Autodesk Inventor part; units mm, degrees
(part 2 of 3)
  point P0 (100, -8.64)
  point P1 (128.2327, 105.01)
  point P2 (153.2327, 105.01)
  point P3 (180, 101.1463)
  point P4 (178.2327, 105.01)
  point P5 (103.2327, 105.01)
  point P6 (8.5673, 105.01)
  point P7 (78.2327, 105.01)
  point P8 (53.2327, 105.01)
  point P9 (28.2327, 105.01)
  point P10 (128.2327, 105.01)
  point P11 (153.2327, 105.01)
  point P12 (178.2327, 105.01)
  point P13 (103.2327, 105.01)
  point P14 (78.2327, 105.01)
  point P15 (53.2327, 105.01)
  point P16 (28.2327, 105.01)
  point P17 (3.2779, 105.049)
  point P18 (3.2327, 105.01)
  point P19 (8.5221, 105.049)
  dimension "d96" = 1.8
  dimension "d97" = 0.9
  dimension "d100" = 25
  constraints: 98 end point, 82 point on circle, 32 centre point, 8 symmetric about line, 2 coincident, 1 horizontal, 1 vertical, 220 other
  measures "d96" distance between parallel lines of L3 L1
  measures "d97" distance between parallel lines of L115 L111
  measures "d100" distance of L0.end L120.start
extrude "Wyciągnięcie proste7" cut sketch "Szkic8" against normal up to surface (1.2 mm away) contours L0 L1 A0 L110 A1 | A3 L116 A2 L3 L4 | L12 L11 A6 L122 A7 | A8 L123 A9 L9 L8 | L33 L32 A10 L128 A11 | A32 L159 A33 L57 L56 | A12 L129 A13 L30 L29 | L55 L54 A14 L134 A15 | L60 L59 A30 L158 A31 | A28 L153 A29 L62 L61 | A16 L135 A17 L52 L51 | L69 L70 A18 L140 A19 | L65 L64 A26 L152 A27 | A24 L147 A25 L46 L47 | A20 L141 A21 L72 L73 | L43 L44 A22 L146 A23
sketch "Szkic9" plane through (-110, 55, 0) normal (0, 1, 0) x (1, 0, 0)
  line L0 (66.3974, -14.0224) -> (153.6026, -14.0224) construction
  line L1 (153.6026, -14.0224) -> (153.6026, -101.2276) construction
  line L2 (153.6026, -101.2276) -> (66.3974, -101.2276) construction
  line L3 (66.3974, -101.2276) -> (66.3974, -14.0224) construction
  line L4 (0, 0) -> (0, -115.25) projected
  line L5 (220, 0) -> (220, -115.25) projected
  line L6 (220, 0) -> (0, 0) projected
  line L7 (220, -115.25) -> (0, -115.25) projected
  point P0 (110, 0)
  dimension "d115" = 66.3975
  dimension "d117" = 87.2051
  dimension "d118" = 220
  dimension "d121" = 115.25
  dimension "d122" = 87.2051
  dimension "d123" = 14.0224
  constraints: 2 other
  measures "d115" distance between parallel lines of L4 L3
  measures "d117" distance between parallel lines of L1 L3
  measures "d118" distance between parallel lines of L5 L4
  measures "d121" distance between parallel lines of L6 L7
  measures "d122" distance between parallel lines of L0 L2
  measures "d123" distance between parallel lines of L6 L0
decal "Pokrycie bitmapą1"
ref_plane "Płaszczyzna konstrukcyjna8" through (-110, 55, 0) normal (0, 1, 0) x (1, 0, 0)
sketch "Szkic13" plane through (-110, 55, 0) normal (0, 1, 0) x (1, 0, 0)
  spline S0 degree 3 poles (103.4764, -89.9857) (102.0188, -89.9857) (101.1686, -88.8719) (101.1686, -87.4139) (101.1686, -85.9559) (102.0188, -84.8422) (103.4764, -84.8422) (104.9341, -84.8422) (105.7843, -85.9559) (105.7843, -87.4139) (105.7843, -88.8719) (104.9341, -89.9857) (103.4764, -89.9857) knots 0 0 0 0 0.25 0.25 0.25 0.5 0.5 0.5 0.75 0.75 0.75 1 1 1 1
  line L0 (103.4764, -89.9857) -> (102.0188, -89.9857) construction
  line L1 (102.0188, -89.9857) -> (101.1686, -88.8719) construction
  line L2 (101.1686, -88.8719) -> (101.1686, -87.4139) construction
  line L3 (101.1686, -87.4139) -> (101.1686, -85.9559) construction
  line L4 (101.1686, -85.9559) -> (102.0188, -84.8422) construction
  line L5 (102.0188, -84.8422) -> (103.4764, -84.8422) construction
  line L6 (103.4764, -84.8422) -> (104.9341, -84.8422) construction
  line L7 (104.9341, -84.8422) -> (105.7843, -85.9559) construction
  line L8 (105.7843, -85.9559) -> (105.7843, -87.4139) construction
  line L9 (105.7843, -87.4139) -> (105.7843, -88.8719) construction
  line L10 (105.7843, -88.8719) -> (104.9341, -89.9857) construction
  line L11 (104.9341, -89.9857) -> (103.4764, -89.9857) construction
  spline S1 degree 3 poles (105.7843, -83.3845) (105.096, -82.7766) (104.2254, -82.3921) (103.1727, -82.3921) (100.3586, -82.3921) (98.5368, -84.5991) (98.5368, -87.4139) (98.5368, -90.2284) (100.3586, -92.4562) (103.1727, -92.4562) (104.2254, -92.4562) (105.096, -92.0713) (105.7843, -91.4638) knots 0 0 0 0 0.111111 0.111111 0.111111 0.222222 0.222222 0.222222 0.333333 0.333333 0.333333 0.444444 0.444444 0.444444 0.444444
  line L12 (105.7843, -83.3845) -> (105.096, -82.7766) construction
  line L13 (105.096, -82.7766) -> (104.2254, -82.3921) construction
  line L14 (104.2254, -82.3921) -> (103.1727, -82.3921) construction
  line L15 (103.1727, -82.3921) -> (100.3586, -82.3921) construction
  line L16 (100.3586, -82.3921) -> (98.5368, -84.5991) construction
  line L17 (98.5368, -84.5991) -> (98.5368, -87.4139) construction
  line L18 (98.5368, -87.4139) -> (98.5368, -90.2284) construction
  line L19 (98.5368, -90.2284) -> (100.3586, -92.4562) construction
  line L20 (100.3586, -92.4562) -> (103.1727, -92.4562) construction
  line L21 (103.1727, -92.4562) -> (104.2254, -92.4562) construction
  line L22 (104.2254, -92.4562) -> (105.096, -92.0713) construction
  line L23 (105.096, -92.0713) -> (105.7843, -91.4638) construction
  line L24 (105.7843, -91.4638) -> (105.7843, -92.2939)
  line L25 (105.7843, -92.2939) -> (108.4767, -92.2939)
  line L26 (108.4767, -92.2939) -> (108.4767, -78.1196)
  line L27 (108.4767, -78.1196) -> (105.7843, -78.1196)
  line L28 (105.7843, -78.1196) -> (105.7843, -83.3845)
  spline S2 degree 3 poles (152.4794, -86.3203) (150.9406, -85.8546) (150.6576, -85.6119) (150.6372, -85.2471) knots 0 0 0 0 0.071429 0.071429 0.071429 0.071429
  line L29 (152.4794, -86.3203) -> (150.9406, -85.8546) construction
  line L30 (150.9406, -85.8546) -> (150.6576, -85.6119) construction
  line L31 (150.6576, -85.6119) -> (150.6372, -85.2471) construction
  spline S3 degree 3 poles (150.6372, -85.2471) (150.6167, -84.984) (150.8802, -84.4781) (151.9125, -84.5589) knots 0.071429 0.071429 0.071429 0.071429 0.142857 0.142857 0.142857 0.142857
  line L32 (150.6372, -85.2471) -> (150.6167, -84.984) construction
  line L33 (150.6167, -84.984) -> (150.8802, -84.4781) construction
  line L34 (150.8802, -84.4781) -> (151.9125, -84.5589) construction
  spline S4 degree 3 poles (151.9125, -84.5589) (152.6614, -84.6195) (152.9853, -85.0852) (153.0865, -85.4091) knots 0.142857 0.142857 0.142857 0.142857 0.214286 0.214286 0.214286 0.214286
  line L35 (151.9125, -84.5589) -> (152.6614, -84.6195) construction
  line L36 (152.6614, -84.6195) -> (152.9853, -85.0852) construction
  line L37 (152.9853, -85.0852) -> (153.0865, -85.4091) construction
  line L38 (153.0865, -85.4091) -> (155.1517, -84.822)
  spline S5 degree 3 poles (155.1517, -84.822) (155.0102, -83.9313) (153.8965, -82.4122) (151.5481, -82.4122) (149.0176, -82.4122) (147.9243, -83.83) (147.8636, -85.1865) knots 0.285714 0.285714 0.285714 0.285714 0.357143 0.357143 0.357143 0.428571 0.428571 0.428571 0.428571
  line L39 (155.1517, -84.822) -> (155.0102, -83.9313) construction
  line L40 (155.0102, -83.9313) -> (153.8965, -82.4122) construction
  line L41 (153.8965, -82.4122) -> (151.5481, -82.4122) construction
  line L42 (151.5481, -82.4122) -> (149.0176, -82.4122) construction
  line L43 (149.0176, -82.4122) -> (147.9243, -83.83) construction
  line L44 (147.9243, -83.83) -> (147.8636, -85.1865) construction
  spline S6 degree 3 poles (147.8636, -85.1865) (147.803, -86.7863) (148.7343, -87.5151) (150.8598, -88.2644) knots 0.428571 0.428571 0.428571 0.428571 0.5 0.5 0.5 0.5
  line L45 (147.8636, -85.1865) -> (147.803, -86.7863) construction
  line L46 (147.803, -86.7863) -> (148.7343, -87.5151) construction
  line L47 (148.7343, -87.5151) -> (150.8598, -88.2644) construction
  spline S7 degree 3 poles (150.8598, -88.2644) (152.2162, -88.7301) (152.6819, -88.7908) (152.7023, -89.3376) knots 0.5 0.5 0.5 0.5 0.571429 0.571429 0.571429 0.571429
  line L48 (150.8598, -88.2644) -> (152.2162, -88.7301) construction
  line L49 (152.2162, -88.7301) -> (152.6819, -88.7908) construction
  line L50 (152.6819, -88.7908) -> (152.7023, -89.3376) construction
  spline S8 degree 3 poles (152.7023, -89.3376) (152.7221, -89.8639) (151.9125, -90.0463) (151.1836, -90.0061) knots 0.571429 0.571429 0.571429 0.571429 0.642857 0.642857 0.642857 0.642857
  line L51 (152.7023, -89.3376) -> (152.7221, -89.8639) construction
  line L52 (152.7221, -89.8639) -> (151.9125, -90.0463) construction
  line L53 (151.9125, -90.0463) -> (151.1836, -90.0061) construction
  spline S9 degree 3 poles (151.1836, -90.0061) (150.4954, -89.9652) (149.6452, -89.5606) (149.4427, -89.054) knots 0.642857 0.642857 0.642857 0.642857 0.714286 0.714286 0.714286 0.714286
  line L54 (151.1836, -90.0061) -> (150.4954, -89.9652) construction
  line L55 (150.4954, -89.9652) -> (149.6452, -89.5606) construction
  line L56 (149.6452, -89.5606) -> (149.4427, -89.054) construction
  line L57 (149.4427, -89.054) -> (147.4788, -90.1074)
  spline S10 degree 3 poles (147.4788, -90.1074) (147.803, -91.3015) (149.6046, -92.4357) (151.6493, -92.4357) (153.8965, -92.4357) (155.4755, -91.2412) (155.5366, -89.4791) knots 0.785714 0.785714 0.785714 0.785714 0.857143 0.857143 0.857143 0.928571 0.928571 0.928571 0.928571
  line L58 (147.4788, -90.1074) -> (147.803, -91.3015) construction
  line L59 (147.803, -91.3015) -> (149.6046, -92.4357) construction
  line L60 (149.6046, -92.4357) -> (151.6493, -92.4357) construction
  line L61 (151.6493, -92.4357) -> (153.8965, -92.4357) construction
  line L62 (153.8965, -92.4357) -> (155.4755, -91.2412) construction
  line L63 (155.4755, -91.2412) -> (155.5366, -89.4791) construction
  spline S11 degree 3 poles (155.5366, -89.4791) (155.5972, -88.0013) (154.7672, -87.029) (152.4794, -86.3203) knots 0.928571 0.928571 0.928571 0.928571 1 1 1 1
  line L64 (155.5366, -89.4791) -> (155.5972, -88.0013) construction
  line L65 (155.5972, -88.0013) -> (154.7672, -87.029) construction
  line L66 (154.7672, -87.029) -> (152.4794, -86.3203) construction
  spline S12 degree 3 poles (141.9948, -89.9857) (140.5372, -89.9857) (139.6866, -88.8719) (139.6866, -87.4139) (139.6866, -85.9559) (140.5372, -84.8422) (141.9948, -84.8422) (143.4321, -84.8422) (144.2822, -85.9559) (144.2822, -87.4139) (144.2822, -88.8719) (143.4321, -89.9857) (141.9948, -89.9857) knots 0 0 0 0 0.25 0.25 0.25 0.5 0.5 0.5 0.75 0.75 0.75 1 1 1 1
  line L67 (141.9948, -89.9857) -> (140.5372, -89.9857) construction
  line L68 (140.5372, -89.9857) -> (139.6866, -88.8719) construction
  line L69 (139.6866, -88.8719) -> (139.6866, -87.4139) construction
  line L70 (139.6866, -87.4139) -> (139.6866, -85.9559) construction
  line L71 (139.6866, -85.9559) -> (140.5372, -84.8422) construction
  line L72 (140.5372, -84.8422) -> (141.9948, -84.8422) construction
  line L73 (141.9948, -84.8422) -> (143.4321, -84.8422) construction
  line L74 (143.4321, -84.8422) -> (144.2822, -85.9559) construction
  line L75 (144.2822, -85.9559) -> (144.2822, -87.4139) construction
  line L76 (144.2822, -87.4139) -> (144.2822, -88.8719) construction
  line L77 (144.2822, -88.8719) -> (143.4321, -89.9857) construction
  line L78 (143.4321, -89.9857) -> (141.9948, -89.9857) construction
  spline S13 degree 3 poles (142.2781, -82.3921) (141.2455, -82.3921) (140.3551, -82.7766) (139.6866, -83.3845) knots 0 0 0 0 0.111111 0.111111 0.111111 0.111111
  line L79 (142.2781, -82.3921) -> (141.2455, -82.3921) construction
  line L80 (141.2455, -82.3921) -> (140.3551, -82.7766) construction
  line L81 (140.3551, -82.7766) -> (139.6866, -83.3845) construction
  line L82 (139.6866, -83.3845) -> (139.6866, -78.1196)
  line L83 (139.6866, -78.1196) -> (136.9942, -78.1196)
  line L84 (136.9942, -78.1196) -> (136.9942, -92.2939)
  line L85 (136.9942, -92.2939) -> (139.6866, -92.2939)
  line L86 (139.6866, -92.2939) -> (139.6866, -91.4638)
  spline S14 degree 3 poles (139.6866, -91.4638) (140.3551, -92.0713) (141.2455, -92.4562) (142.2781, -92.4562) (145.0922, -92.4562) (146.9746, -90.2284) (146.9746, -87.4139) (146.9746, -84.5991) (145.0922, -82.3921) (142.2781, -82.3921) knots 0.666667 0.666667 0.666667 0.666667 0.777778 0.777778 0.777778 0.888889 0.888889 0.888889 1 1 1 1
  line L87 (139.6866, -91.4638) -> (140.3551, -92.0713) construction
  line L88 (140.3551, -92.0713) -> (141.2455, -92.4562) construction
  line L89 (141.2455, -92.4562) -> (142.2781, -92.4562) construction
  line L90 (142.2781, -92.4562) -> (145.0922, -92.4562) construction
  line L91 (145.0922, -92.4562) -> (146.9746, -90.2284) construction
  line L92 (146.9746, -90.2284) -> (146.9746, -87.4139) construction
  line L93 (146.9746, -87.4139) -> (146.9746, -84.5991) construction
  line L94 (146.9746, -84.5991) -> (145.0922, -82.3921) construction
  line L95 (145.0922, -82.3921) -> (142.2781, -82.3921) construction
  spline S15 degree 3 poles (123.5872, -89.9652) (122.8584, -89.9049) (122.6965, -89.1757) (122.6965, -88.5075) knots 0 0 0 0 0.125 0.125 0.125 0.125
  line L96 (123.5872, -89.9652) -> (122.8584, -89.9049) construction
  line L97 (122.8584, -89.9049) -> (122.6965, -89.1757) construction
  line L98 (122.6965, -89.1757) -> (122.6965, -88.5075) construction
  line L99 (122.6965, -88.5075) -> (122.6965, -77.1071)
  line L100 (122.6965, -77.1071) -> (120.0037, -77.1071)
  line L101 (120.0037, -77.1071) -> (120.0037, -88.3657)
  spline S16 degree 3 poles (120.0037, -88.3657) (120.0037, -91.6056) (121.2593, -92.375) (122.9191, -92.4562) knots 0.5 0.5 0.5 0.5 0.625 0.625 0.625 0.625
  line L102 (120.0037, -88.3657) -> (120.0037, -91.6056) construction
  line L103 (120.0037, -91.6056) -> (121.2593, -92.375) construction
  line L104 (121.2593, -92.375) -> (122.9191, -92.4562) construction
  spline S17 degree 3 poles (122.9191, -92.4562) (124.0935, -92.5168) (125.8125, -92.36) (125.8143, -92.3598) knots 0.625 0.625 0.625 0.625 0.75 0.75 0.75 0.75
  line L105 (122.9191, -92.4562) -> (124.0935, -92.5168) construction
  line L106 (124.0935, -92.5168) -> (125.8143, -92.3598) construction
  line L107 (125.8143, -92.3598) -> (125.8143, -92.3598) construction
  line L108 (125.8143, -92.3598) -> (125.6171, -89.9941)
  spline S18 degree 3 poles (125.6171, -89.9941) (125.6155, -89.9942) (124.0123, -90.0061) (123.5872, -89.9652) knots 0.875 0.875 0.875 0.875 1 1 1 1
  line L109 (125.6171, -89.9941) -> (125.6171, -89.9941) construction
  line L110 (125.6171, -89.9941) -> (124.0123, -90.0061) construction
  line L111 (124.0123, -90.0061) -> (123.5872, -89.9652) construction
  spline S19 degree 3 poles (112.443, -86.5027) (112.6857, -85.5308) (113.3944, -84.8422) (114.5283, -84.8422) (115.6617, -84.8422) (116.2689, -85.5308) (116.4918, -86.5027) knots 0 0 0 0 0.333333 0.333333 0.333333 0.666667 0.666667 0.666667 0.666667
  line L112 (112.443, -86.5027) -> (112.6857, -85.5308) construction
  line L113 (112.6857, -85.5308) -> (113.3944, -84.8422) construction
  line L114 (113.3944, -84.8422) -> (114.5283, -84.8422) construction
  line L115 (114.5283, -84.8422) -> (115.6617, -84.8422) construction
  line L116 (115.6617, -84.8422) -> (116.2689, -85.5308) construction
  line L117 (116.2689, -85.5308) -> (116.4918, -86.5027) construction
  line L118 (116.4918, -86.5027) -> (112.443, -86.5027)
  spline S20 degree 3 poles (114.5283, -82.3921) (111.7138, -82.3921) (109.6896, -84.5991) (109.6896, -87.4139) (109.6896, -90.2284) (111.815, -92.4562) (114.6292, -92.4562) (116.411, -92.4562) (117.8483, -91.565) (118.6579, -90.2083) knots 0 0 0 0 0.111111 0.111111 0.111111 0.222222 0.222222 0.222222 0.333333 0.333333 0.333333 0.333333
  line L119 (114.5283, -82.3921) -> (111.7138, -82.3921) construction
  line L120 (111.7138, -82.3921) -> (109.6896, -84.5991) construction
  line L121 (109.6896, -84.5991) -> (109.6896, -87.4139) construction
  line L122 (109.6896, -87.4139) -> (109.6896, -90.2284) construction
  line L123 (109.6896, -90.2284) -> (111.815, -92.4562) construction
  line L124 (111.815, -92.4562) -> (114.6292, -92.4562) construction
  line L125 (114.6292, -92.4562) -> (116.411, -92.4562) construction
  line L126 (116.411, -92.4562) -> (117.8483, -91.565) construction
  line L127 (117.8483, -91.565) -> (118.6579, -90.2083) construction
  line L128 (118.6579, -90.2083) -> (116.4308, -89.1146)
  spline S21 degree 3 poles (116.4308, -89.1146) (116.0463, -89.6614) (115.4187, -89.9857) (114.6292, -89.9857) (113.5158, -89.9857) (112.7665, -89.3376) (112.4631, -88.3858) knots 0.444444 0.444444 0.444444 0.444444 0.555556 0.555556 0.555556 0.666667 0.666667 0.666667 0.666667
  line L129 (116.4308, -89.1146) -> (116.0463, -89.6614) construction
  line L130 (116.0463, -89.6614) -> (115.4187, -89.9857) construction
  line L131 (115.4187, -89.9857) -> (114.6292, -89.9857) construction
  line L132 (114.6292, -89.9857) -> (113.5158, -89.9857) construction
  line L133 (113.5158, -89.9857) -> (112.7665, -89.3376) construction
  line L134 (112.7665, -89.3376) -> (112.4631, -88.3858) construction
  line L135 (112.4631, -88.3858) -> (118.9616, -88.3858)
  spline S22 degree 3 poles (118.9616, -88.3858) (119.0223, -88.0821) (119.0428, -87.7582) (119.0428, -87.4139) (119.0428, -84.5991) (117.3219, -82.3921) (114.5283, -82.3921) knots 0.777778 0.777778 0.777778 0.777778 0.888889 0.888889 0.888889 1 1 1 1
  line L136 (118.9616, -88.3858) -> (119.0223, -88.0821) construction
  line L137 (119.0223, -88.0821) -> (119.0428, -87.7582) construction
  line L138 (119.0428, -87.7582) -> (119.0428, -87.4139) construction
  line L139 (119.0428, -87.4139) -> (119.0428, -84.5991) construction
  line L140 (119.0428, -84.5991) -> (117.3219, -82.3921) construction
  line L141 (117.3219, -82.3921) -> (114.5283, -82.3921) construction
  spline S23 degree 3 poles (83.196, -88.3047) (83.1148, -89.3782) (82.3659, -90.2083) (81.3132, -90.3705) knots 0 0 0 0 0.2 0.2 0.2 0.2
  line L142 (83.196, -88.3047) -> (83.1148, -89.3782) construction
  line L143 (83.1148, -89.3782) -> (82.3659, -90.2083) construction
  line L144 (82.3659, -90.2083) -> (81.3132, -90.3705) construction
  spline S24 degree 3 poles (81.3132, -90.3705) (80.7057, -90.4718) (80.0982, -90.3501) (79.9363, -89.9049) knots 0.2 0.2 0.2 0.2 0.4 0.4 0.4 0.4
  line L145 (81.3132, -90.3705) -> (80.7057, -90.4718) construction
  line L146 (80.7057, -90.4718) -> (80.0982, -90.3501) construction
  line L147 (80.0982, -90.3501) -> (79.9363, -89.9049) construction
  spline S25 degree 3 poles (79.9363, -89.9049) (79.7543, -89.4187) (80.0375, -88.7707) (81.0295, -88.5075) knots 0.4 0.4 0.4 0.4 0.6 0.6 0.6 0.6
  line L148 (79.9363, -89.9049) -> (79.7543, -89.4187) construction
  line L149 (79.7543, -89.4187) -> (80.0375, -88.7707) construction
  line L150 (80.0375, -88.7707) -> (81.0295, -88.5075) construction
  spline S26 degree 3 poles (81.0295, -88.5075) (82.3048, -88.1837) (83.1951, -88.0015) (83.196, -88.0013) knots 0.6 0.6 0.6 0.6 0.8 0.8 0.8 0.8
  line L151 (81.0295, -88.5075) -> (82.3048, -88.1837) construction
  line L152 (82.3048, -88.1837) -> (83.196, -88.0013) construction
  line L153 (83.196, -88.0013) -> (83.196, -88.0013) construction
  line L154 (83.196, -88.0013) -> (83.196, -88.3047)
  spline S27 degree 3 poles (81.8797, -82.3921) (79.4505, -82.3921) (78.0129, -83.992) (77.8309, -85.2676) knots 0 0 0 0 0.083333 0.083333 0.083333 0.083333
  line L155 (81.8797, -82.3921) -> (79.4505, -82.3921) construction
  line L156 (79.4505, -82.3921) -> (78.0129, -83.992) construction
  line L157 (78.0129, -83.992) -> (77.8309, -85.2676) construction
  line L158 (77.8309, -85.2676) -> (80.0781, -85.7537)
  spline S28 degree 3 poles (80.0781, -85.7537) (80.24, -85.0044) (80.8676, -84.6195) (81.6977, -84.5991) knots 0.166667 0.166667 0.166667 0.166667 0.25 0.25 0.25 0.25
  line L159 (80.0781, -85.7537) -> (80.24, -85.0044) construction
  line L160 (80.24, -85.0044) -> (80.8676, -84.6195) construction
  line L161 (80.8676, -84.6195) -> (81.6977, -84.5991) construction
  spline S29 degree 3 poles (81.6977, -84.5991) (82.6491, -84.5589) (83.2767, -85.1664) (83.1349, -85.7537) knots 0.25 0.25 0.25 0.25 0.333333 0.333333 0.333333 0.333333
  line L162 (81.6977, -84.5991) -> (82.6491, -84.5589) construction
  line L163 (82.6491, -84.5589) -> (83.2767, -85.1664) construction
  line L164 (83.2767, -85.1664) -> (83.1349, -85.7537) construction
  spline S30 degree 3 poles (83.1349, -85.7537) (83.0136, -86.3002) (82.3253, -86.3002) (80.6856, -86.6646) knots 0.333333 0.333333 0.333333 0.333333 0.416667 0.416667 0.416667 0.416667
  line L165 (83.1349, -85.7537) -> (83.0136, -86.3002) construction
  line L166 (83.0136, -86.3002) -> (82.3253, -86.3002) construction
  line L167 (82.3253, -86.3002) -> (80.6856, -86.6646) construction
  spline S31 degree 3 poles (80.6856, -86.6646) (78.6204, -87.1105) (77.1627, -87.8595) (77.1627, -89.9857) knots 0.416667 0.416667 0.416667 0.416667 0.5 0.5 0.5 0.5
  line L168 (80.6856, -86.6646) -> (78.6204, -87.1105) construction
  line L169 (78.6204, -87.1105) -> (77.1627, -87.8595) construction
  line L170 (77.1627, -87.8595) -> (77.1627, -89.9857) construction
  spline S32 degree 3 poles (77.1627, -89.9857) (77.2439, -91.4638) (78.2966, -92.4562) (80.1995, -92.4562) (81.8596, -92.4562) (82.8315, -91.7471) (83.196, -91.3827) knots 0.5 0.5 0.5 0.5 0.583333 0.583333 0.583333 0.666667 0.666667 0.666667 0.666667
  line L171 (77.1627, -89.9857) -> (77.2439, -91.4638) construction
  line L172 (77.2439, -91.4638) -> (78.2966, -92.4562) construction
  line L173 (78.2966, -92.4562) -> (80.1995, -92.4562) construction
  line L174 (80.1995, -92.4562) -> (81.8596, -92.4562) construction
  line L175 (81.8596, -92.4562) -> (82.8315, -91.7471) construction
  line L176 (82.8315, -91.7471) -> (83.196, -91.3827) construction
  line L177 (83.196, -91.3827) -> (83.196, -92.2939)
  line L178 (83.196, -92.2939) -> (85.8679, -92.2939)
  line L179 (85.8679, -92.2939) -> (85.8679, -86.1993)
  spline S33 degree 3 poles (85.8679, -86.1993) (85.8679, -83.364) (84.0056, -82.3921) (81.8797, -82.3921) knots 0.916667 0.916667 0.916667 0.916667 1 1 1 1
  line L180 (85.8679, -86.1993) -> (85.8679, -83.364) construction
  line L181 (85.8679, -83.364) -> (84.0056, -82.3921) construction
  line L182 (84.0056, -82.3921) -> (81.8797, -82.3921) construction
  line L183 (73.1478, -83.8678) -> (67.5033, -83.8678)
  line L184 (67.5033, -83.8678) -> (67.5033, -78.2233)
  line L185 (67.5033, -78.2233) -> (64.6811, -78.2233)
  line L186 (64.6811, -78.2233) -> (64.6811, -83.8678)
  line L187 (64.6811, -83.8678) -> (64.6811, -86.69)
  line L188 (64.6811, -86.69) -> (64.6811, -92.3344)
  line L189 (64.6811, -92.3344) -> (67.5033, -92.3344)
  line L190 (67.5033, -92.3344) -> (67.5033, -86.69)
  line L191 (67.5033, -86.69) -> (73.1478, -86.69)
  line L192 (73.1478, -86.69) -> (73.1478, -92.3344)
  line L193 (73.1478, -92.3344) -> (75.97, -92.3344)
  line L194 (75.97, -92.3344) -> (75.97, -86.69)
  line L195 (75.97, -86.69) -> (75.97, -83.8678)
  line L196 (75.97, -83.8678) -> (75.97, -78.2233)
  line L197 (75.97, -78.2233) -> (73.1478, -78.2233)
  line L198 (73.1478, -78.2233) -> (73.1478, -83.8678)
  spline S34 degree 3 poles (132.7041, -88.3047) (132.6233, -89.3782) (131.8743, -90.2083) (130.8213, -90.3705) knots 0 0 0 0 0.2 0.2 0.2 0.2
  line L199 (132.7041, -88.3047) -> (132.6233, -89.3782) construction
  line L200 (132.6233, -89.3782) -> (131.8743, -90.2083) construction
  line L201 (131.8743, -90.2083) -> (130.8213, -90.3705) construction
  spline S35 degree 3 poles (130.8213, -90.3705) (130.2142, -90.4718) (129.6067, -90.3501) (129.4448, -89.9049) knots 0.2 0.2 0.2 0.2 0.4 0.4 0.4 0.4
  line L202 (130.8213, -90.3705) -> (130.2142, -90.4718) construction
  line L203 (130.2142, -90.4718) -> (129.6067, -90.3501) construction
  line L204 (129.6067, -90.3501) -> (129.4448, -89.9049) construction
  spline S36 degree 3 poles (129.4448, -89.9049) (129.2627, -89.4187) (129.546, -88.7707) (130.538, -88.5075) knots 0.4 0.4 0.4 0.4 0.6 0.6 0.6 0.6
  line L205 (129.4448, -89.9049) -> (129.2627, -89.4187) construction
  line L206 (129.2627, -89.4187) -> (129.546, -88.7707) construction
  line L207 (129.546, -88.7707) -> (130.538, -88.5075) construction
  spline S37 degree 3 poles (130.538, -88.5075) (131.8137, -88.1837) (132.7032, -88.0015) (132.7041, -88.0013) knots 0.6 0.6 0.6 0.6 0.8 0.8 0.8 0.8
  line L208 (130.538, -88.5075) -> (131.8137, -88.1837) construction
  line L209 (131.8137, -88.1837) -> (132.7041, -88.0013) construction
  line L210 (132.7041, -88.0013) -> (132.7041, -88.0013) construction
  line L211 (132.7041, -88.0013) -> (132.7041, -88.3047)
  spline S38 degree 3 poles (131.3886, -82.3921) (128.959, -82.3921) (127.5218, -83.992) (127.3394, -85.2676) knots 0 0 0 0 0.083333 0.083333 0.083333 0.083333
  line L212 (131.3886, -82.3921) -> (128.959, -82.3921) construction
  line L213 (128.959, -82.3921) -> (127.5218, -83.992) construction
  line L214 (127.5218, -83.992) -> (127.3394, -85.2676) construction
  line L215 (127.3394, -85.2676) -> (129.5866, -85.7537)
  spline S39 degree 3 poles (129.5866, -85.7537) (129.7485, -85.0044) (130.3761, -84.6195) (131.2062, -84.5991) knots 0.166667 0.166667 0.166667 0.166667 0.25 0.25 0.25 0.25
  line L216 (129.5866, -85.7537) -> (129.7485, -85.0044) construction
  line L217 (129.7485, -85.0044) -> (130.3761, -84.6195) construction
  line L218 (130.3761, -84.6195) -> (131.2062, -84.5991) construction
  spline S40 degree 3 poles (131.2062, -84.5991) (132.1576, -84.5589) (132.7852, -85.1664) (132.6434, -85.7537) knots 0.25 0.25 0.25 0.25 0.333333 0.333333 0.333333 0.333333
  line L219 (131.2062, -84.5991) -> (132.1576, -84.5589) construction
  line L220 (132.1576, -84.5589) -> (132.7852, -85.1664) construction
  line L221 (132.7852, -85.1664) -> (132.6434, -85.7537) construction
  spline S41 degree 3 poles (132.6434, -85.7537) (132.522, -86.3002) (131.8338, -86.3002) (130.1941, -86.6646) knots 0.333333 0.333333 0.333333 0.333333 0.416667 0.416667 0.416667 0.416667
  line L222 (132.6434, -85.7537) -> (132.522, -86.3002) construction
  line L223 (132.522, -86.3002) -> (131.8338, -86.3002) construction
  line L224 (131.8338, -86.3002) -> (130.1941, -86.6646) construction
  spline S42 degree 3 poles (130.1941, -86.6646) (128.1289, -87.1105) (126.6716, -87.8595) (126.6716, -89.9857) knots 0.416667 0.416667 0.416667 0.416667 0.5 0.5 0.5 0.5
  line L225 (130.1941, -86.6646) -> (128.1289, -87.1105) construction
  line L226 (128.1289, -87.1105) -> (126.6716, -87.8595) construction
  line L227 (126.6716, -87.8595) -> (126.6716, -89.9857) construction
  spline S43 degree 3 poles (126.6716, -89.9857) (126.7524, -91.4638) (127.8047, -92.4562) (129.7079, -92.4562) (131.3681, -92.4562) (132.34, -91.7471) (132.7041, -91.3827) knots 0.5 0.5 0.5 0.5 0.583333 0.583333 0.583333 0.666667 0.666667 0.666667 0.666667
  line L228 (126.6716, -89.9857) -> (126.7524, -91.4638) construction
  line L229 (126.7524, -91.4638) -> (127.8047, -92.4562) construction
  line L230 (127.8047, -92.4562) -> (129.7079, -92.4562) construction
  line L231 (129.7079, -92.4562) -> (131.3681, -92.4562) construction
  line L232 (131.3681, -92.4562) -> (132.34, -91.7471) construction
  line L233 (132.34, -91.7471) -> (132.7041, -91.3827) construction
  line L234 (132.7041, -91.3827) -> (132.7041, -92.2939)
  line L235 (132.7041, -92.2939) -> (135.3764, -92.2939)
  line L236 (135.3764, -92.2939) -> (135.3764, -86.1993)
  spline S44 degree 3 poles (135.3764, -86.1993) (135.3764, -83.364) (133.5141, -82.3921) (131.3886, -82.3921) knots 0.916667 0.916667 0.916667 0.916667 1 1 1 1
  line L237 (135.3764, -86.1993) -> (135.3764, -83.364) construction
  line L238 (135.3764, -83.364) -> (133.5141, -82.3921) construction
  line L239 (133.5141, -82.3921) -> (131.3886, -82.3921) construction
  line L240 (94.4683, -92.2939) -> (97.161, -92.2939)
  line L241 (97.161, -92.2939) -> (97.161, -82.5339)
  line L242 (97.161, -82.5339) -> (94.4683, -82.5339)
  line L243 (94.4683, -82.5339) -> (94.4683, -92.2939)
  spline S45 degree 3 poles (95.825, -78.1602) (94.9745, -78.1602) (94.3063, -78.8283) (94.3063, -79.6785) (94.3063, -80.509) (94.9745, -81.1771) (95.825, -81.1771) (96.6551, -81.1771) (97.3229, -80.509) (97.3229, -79.6785) (97.3229, -78.8283) (96.6551, -78.1602) (95.825, -78.1602) knots 0 0 0 0 0.25 0.25 0.25 0.5 0.5 0.5 0.75 0.75 0.75 1 1 1 1
  line L244 (95.825, -78.1602) -> (94.9745, -78.1602) construction
  line L245 (94.9745, -78.1602) -> (94.3063, -78.8283) construction
  line L246 (94.3063, -78.8283) -> (94.3063, -79.6785) construction
  line L247 (94.3063, -79.6785) -> (94.3063, -80.509) construction
  line L248 (94.3063, -80.509) -> (94.9745, -81.1771) construction
  line L249 (94.9745, -81.1771) -> (95.825, -81.1771) construction
  line L250 (95.825, -81.1771) -> (96.6551, -81.1771) construction
  line L251 (96.6551, -81.1771) -> (97.3229, -80.509) construction
  line L252 (97.3229, -80.509) -> (97.3229, -79.6785) construction
  line L253 (97.3229, -79.6785) -> (97.3229, -78.8283) construction
  line L254 (97.3229, -78.8283) -> (96.6551, -78.1602) construction
  line L255 (96.6551, -78.1602) -> (95.825, -78.1602) construction
  spline S46 degree 3 poles (91.1701, -89.9652) (90.4413, -89.9049) (90.2794, -89.1757) (90.2794, -88.5075) knots 0 0 0 0 0.125 0.125 0.125 0.125
  line L256 (91.1701, -89.9652) -> (90.4413, -89.9049) construction
  line L257 (90.4413, -89.9049) -> (90.2794, -89.1757) construction
  line L258 (90.2794, -89.1757) -> (90.2794, -88.5075) construction
  line L259 (90.2794, -88.5075) -> (90.2794, -77.1071)
  line L260 (90.2794, -77.1071) -> (87.587, -77.1071)
  line L261 (87.587, -77.1071) -> (87.587, -88.3657)
  spline S47 degree 3 poles (87.587, -88.3657) (87.587, -91.6056) (88.8422, -92.375) (90.5023, -92.4562) knots 0.5 0.5 0.5 0.5 0.625 0.625 0.625 0.625
  line L262 (87.587, -88.3657) -> (87.587, -91.6056) construction
  line L263 (87.587, -91.6056) -> (88.8422, -92.375) construction
  line L264 (88.8422, -92.375) -> (90.5023, -92.4562) construction
  spline S48 degree 3 poles (90.5023, -92.4562) (91.6764, -92.5168) (93.3954, -92.36) (93.3972, -92.3598) knots 0.625 0.625 0.625 0.625 0.75 0.75 0.75 0.75
  line L265 (90.5023, -92.4562) -> (91.6764, -92.5168) construction
  line L266 (91.6764, -92.5168) -> (93.3972, -92.3598) construction
  line L267 (93.3972, -92.3598) -> (93.3972, -92.3598) construction
  line L268 (93.3972, -92.3598) -> (93.2004, -89.9941)
  spline S49 degree 3 poles (93.2004, -89.9941) (92.9979, -90.1765) (91.5956, -90.0061) (91.1701, -89.9652) knots 0.875 0.875 0.875 0.875 1 1 1 1
  line L269 (93.2004, -89.9941) -> (92.9979, -90.1765) construction
  line L270 (92.9979, -90.1765) -> (91.5956, -90.0061) construction
  line L271 (91.5956, -90.0061) -> (91.1701, -89.9652) construction
  spline S50 degree 3 poles (127.3225, -30.7663) (127.502, -30.4092) (128.3159, -30.3563) (129.5668, -30.4145) knots 0 0 0 0 0.017241 0.017241 0.017241 0.017241
  line L272 (127.3225, -30.7663) -> (127.502, -30.4092) construction
  line L273 (127.502, -30.4092) -> (128.3159, -30.3563) construction
  line L274 (128.3159, -30.3563) -> (129.5668, -30.4145) construction
  spline S51 degree 3 poles (129.5668, -30.4145) (130.8171, -30.4727) (130.7177, -29.7848) (130.7176, -29.7841) knots 0.017241 0.017241 0.017241 0.017241 0.034483 0.034483 0.034483 0.034483
  line L275 (129.5668, -30.4145) -> (130.8171, -30.4727) construction
  line L276 (130.8171, -30.4727) -> (130.7176, -29.7841) construction
  line L277 (130.7176, -29.7841) -> (130.7176, -29.7841) construction
  spline S52 degree 3 poles (130.7176, -29.7841) (131.3755, -29.8452) (131.4344, -29.1735) (131.3113, -28.9643) knots 0.034483 0.034483 0.034483 0.034483 0.051724 0.051724 0.051724 0.051724
  line L278 (130.7176, -29.7841) -> (131.3755, -29.8452) construction
  line L279 (131.3755, -29.8452) -> (131.4344, -29.1735) construction
  line L280 (131.4344, -29.1735) -> (131.3113, -28.9643) construction
  spline S53 degree 3 poles (131.3113, -28.9643) (131.1878, -28.7554) (131.3866, -28.3681) (131.3868, -28.3677) knots 0.051724 0.051724 0.051724 0.051724 0.068966 0.068966 0.068966 0.068966
  line L281 (131.3113, -28.9643) -> (131.1878, -28.7554) construction
  line L282 (131.1878, -28.7554) -> (131.3868, -28.3677) construction
  line L283 (131.3868, -28.3677) -> (131.3868, -28.3677) construction
  spline S54 degree 3 poles (131.3868, -28.3677) (131.7622, -27.7292) (131.0305, -27.4483) (131.0298, -27.448) knots 0.068966 0.068966 0.068966 0.068966 0.086207 0.086207 0.086207 0.086207
  line L284 (131.3868, -28.3677) -> (131.7622, -27.7292) construction
  line L285 (131.7622, -27.7292) -> (131.0298, -27.448) construction
  line L286 (131.0298, -27.448) -> (131.0298, -27.448) construction
  spline S55 degree 3 poles (131.0298, -27.448) (130.5236, -26.9044) (129.1561, -26.1891) (129.1548, -26.1883) knots 0.086207 0.086207 0.086207 0.086207 0.103448 0.103448 0.103448 0.103448
  line L287 (131.0298, -27.448) -> (130.5236, -26.9044) construction
  line L288 (130.5236, -26.9044) -> (129.1548, -26.1883) construction
  line L289 (129.1548, -26.1883) -> (129.1548, -26.1883) construction
  spline S56 degree 3 poles (129.1548, -26.1883) (129.9316, -25.6164) (129.5999, -24.9288) (129.5996, -24.9281) knots 0.103448 0.103448 0.103448 0.103448 0.12069 0.12069 0.12069 0.12069
  line L290 (129.1548, -26.1883) -> (129.9316, -25.6164) construction
  line L291 (129.9316, -25.6164) -> (129.5996, -24.9281) construction
  line L292 (129.5996, -24.9281) -> (129.5996, -24.9281) construction
  spline S57 degree 3 poles (129.5996, -24.9281) (129.3054, -23.7044) (127.2825, -22.8219) (127.2805, -22.821) knots 0.12069 0.12069 0.12069 0.12069 0.137931 0.137931 0.137931 0.137931
  line L293 (129.5996, -24.9281) -> (129.3054, -23.7044) construction
  line L294 (129.3054, -23.7044) -> (127.2805, -22.821) construction
  line L295 (127.2805, -22.821) -> (127.2805, -22.821) construction
  line L296 (127.2805, -22.821) -> (127.4763, -22.3024)
  spline S58 degree 3 poles (127.4763, -22.3024) (127.4769, -22.3008) (128.0845, -20.6101) (128.1984, -20.1893) knots 0.155172 0.155172 0.155172 0.155172 0.172414 0.172414 0.172414 0.172414
  line L297 (127.4763, -22.3024) -> (127.4763, -22.3024) construction
  line L298 (127.4763, -22.3024) -> (128.0845, -20.6101) construction
  line L299 (128.0845, -20.6101) -> (128.1984, -20.1893) construction
  spline S59 degree 3 poles (128.1984, -20.1893) (128.3123, -19.7681) (128.0093, -19.6792) (127.7222, -19.6654) knots 0.172414 0.172414 0.172414 0.172414 0.189655 0.189655 0.189655 0.189655
  line L300 (128.1984, -20.1893) -> (128.3123, -19.7681) construction
  line L301 (128.3123, -19.7681) -> (128.0093, -19.6792) construction
  line L302 (128.0093, -19.6792) -> (127.7222, -19.6654) construction
  spline S60 degree 3 poles (127.7222, -19.6654) (127.4357, -19.6513) (127.3867, -19.6626) (126.812, -20.4517) knots 0.189655 0.189655 0.189655 0.189655 0.206897 0.206897 0.206897 0.206897
  line L303 (127.7222, -19.6654) -> (127.4357, -19.6513) construction
  line L304 (127.4357, -19.6513) -> (127.3867, -19.6626) construction
  line L305 (127.3867, -19.6626) -> (126.812, -20.4517) construction
  spline S61 degree 3 poles (126.812, -20.4517) (126.237, -21.2409) (124.9978, -22.2855) (124.9966, -22.2865) knots 0.206897 0.206897 0.206897 0.206897 0.224138 0.224138 0.224138 0.224138
  line L306 (126.812, -20.4517) -> (126.237, -21.2409) construction
  line L307 (126.237, -21.2409) -> (124.9966, -22.2865) construction
  line L308 (124.9966, -22.2865) -> (124.9966, -22.2865) construction
  spline S62 degree 3 poles (124.9966, -22.2865) (124.9969, -22.2858) (125.2957, -21.5337) (125.4531, -21.0765) knots 0.224138 0.224138 0.224138 0.224138 0.241379 0.241379 0.241379 0.241379
  line L309 (124.9966, -22.2865) -> (124.9966, -22.2865) construction
  line L310 (124.9966, -22.2865) -> (125.2957, -21.5337) construction
  line L311 (125.2957, -21.5337) -> (125.4531, -21.0765) construction
  spline S63 degree 3 poles (125.4531, -21.0765) (125.6108, -20.6193) (125.5469, -20.2122) (125.228, -20.2849) knots 0.241379 0.241379 0.241379 0.241379 0.258621 0.258621 0.258621 0.258621
  line L312 (125.4531, -21.0765) -> (125.6108, -20.6193) construction
  line L313 (125.6108, -20.6193) -> (125.5469, -20.2122) construction
  line L314 (125.5469, -20.2122) -> (125.228, -20.2849) construction
  spline S64 degree 3 poles (125.228, -20.2849) (124.9084, -20.3572) (124.3175, -21.0712) (124.0776, -21.3891) knots 0.258621 0.258621 0.258621 0.258621 0.275862 0.275862 0.275862 0.275862
  line L315 (125.228, -20.2849) -> (124.9084, -20.3572) construction
  line L316 (124.9084, -20.3572) -> (124.3175, -21.0712) construction
  line L317 (124.3175, -21.0712) -> (124.0776, -21.3891) construction
  spline S65 degree 3 poles (124.0776, -21.3891) (123.8377, -21.7069) (122.537, -22.4767) (121.4924, -23.2408) knots 0.275862 0.275862 0.275862 0.275862 0.293103 0.293103 0.293103 0.293103
  line L318 (124.0776, -21.3891) -> (123.8377, -21.7069) construction
  line L319 (123.8377, -21.7069) -> (122.537, -22.4767) construction
  line L320 (122.537, -22.4767) -> (121.4924, -23.2408) construction
  spline S66 degree 3 poles (121.4924, -23.2408) (120.4482, -24.0049) (119.8838, -25.8979) (119.8175, -26.8878) knots 0.293103 0.293103 0.293103 0.293103 0.310345 0.310345 0.310345 0.310345
  line L321 (121.4924, -23.2408) -> (120.4482, -24.0049) construction
  line L322 (120.4482, -24.0049) -> (119.8838, -25.8979) construction
  line L323 (119.8838, -25.8979) -> (119.8175, -26.8878) construction
  spline S67 degree 3 poles (119.8175, -26.8878) (119.7508, -27.8774) (119.3726, -31.2) (119.3723, -31.2033) knots 0.310345 0.310345 0.310345 0.310345 0.327586 0.327586 0.327586 0.327586
  line L324 (119.8175, -26.8878) -> (119.7508, -27.8774) construction
  line L325 (119.7508, -27.8774) -> (119.3723, -31.2033) construction
  line L326 (119.3723, -31.2033) -> (119.3723, -31.2033) construction
  line L327 (119.3723, -31.2033) -> (119.356, -31.3649)
  spline S68 degree 3 poles (119.356, -31.3649) (119.3514, -31.4831) (119.2968, -31.8913) (119.2223, -32.406) knots 0.344828 0.344828 0.344828 0.344828 0.362069 0.362069 0.362069 0.362069
  line L328 (119.356, -31.3649) -> (119.3514, -31.4831) construction
  line L329 (119.3514, -31.4831) -> (119.2968, -31.8913) construction
  line L330 (119.2968, -31.8913) -> (119.2223, -32.406) construction
  spline S69 degree 3 poles (119.2223, -32.406) (118.9048, -33.5567) (118.0984, -35.6854) (117.5625, -38.4773) knots 0.362069 0.362069 0.362069 0.362069 0.37931 0.37931 0.37931 0.37931
  line L331 (119.2223, -32.406) -> (118.9048, -33.5567) construction
  line L332 (118.9048, -33.5567) -> (118.0984, -35.6854) construction
  line L333 (118.0984, -35.6854) -> (117.5625, -38.4773) construction
  spline S70 degree 3 poles (117.5625, -38.4773) (116.9384, -41.7324) (114.5218, -40.622) (114.5194, -40.6208) knots 0.37931 0.37931 0.37931 0.37931 0.396552 0.396552 0.396552 0.396552
  line L334 (117.5625, -38.4773) -> (116.9384, -41.7324) construction
  line L335 (116.9384, -41.7324) -> (114.5194, -40.6208) construction
  line L336 (114.5194, -40.6208) -> (114.5194, -40.6208) construction
  spline S71 degree 3 poles (114.5194, -40.6208) (114.5163, -40.6201) (111.476, -39.827) (110.774, -39.9064) knots 0.396552 0.396552 0.396552 0.396552 0.413793 0.413793 0.413793 0.413793
  line L337 (114.5194, -40.6208) -> (114.5194, -40.6208) construction
  line L338 (114.5194, -40.6208) -> (111.476, -39.827) construction
  line L339 (111.476, -39.827) -> (110.774, -39.9064) construction
  spline S72 degree 3 poles (110.774, -39.9064) (110.0716, -39.9858) (109.4673, -40.4398) (104.1612, -39.09) knots 0.413793 0.413793 0.413793 0.413793 0.431034 0.431034 0.431034 0.431034
  line L340 (110.774, -39.9064) -> (110.0716, -39.9858) construction
  line L341 (110.0716, -39.9858) -> (109.4673, -40.4398) construction
  line L342 (109.4673, -40.4398) -> (104.1612, -39.09) construction
  spline S73 degree 3 poles (104.1612, -39.09) (98.8551, -37.7403) (92.9245, -38.8519) (90.1157, -42.186) knots 0.431034 0.431034 0.431034 0.431034 0.448276 0.448276 0.448276 0.448276
  line L343 (104.1612, -39.09) -> (98.8551, -37.7403) construction
  line L344 (98.8551, -37.7403) -> (92.9245, -38.8519) construction
  line L345 (92.9245, -38.8519) -> (90.1157, -42.186) construction
  spline S74 degree 3 poles (90.1157, -42.186) (88.1535, -44.5147) (88.2858, -46.4945) (88.8362, -47.8827) knots 0.448276 0.448276 0.448276 0.448276 0.465517 0.465517 0.465517 0.465517
  line L346 (90.1157, -42.186) -> (88.1535, -44.5147) construction
  line L347 (88.1535, -44.5147) -> (88.2858, -46.4945) construction
  line L348 (88.2858, -46.4945) -> (88.8362, -47.8827) construction
  spline S75 degree 3 poles (88.8362, -47.8827) (88.8425, -47.8393) (88.8492, -47.7973) (88.8549, -47.7497) knots 0.465517 0.465517 0.465517 0.465517 0.482759 0.482759 0.482759 0.482759
  line L349 (88.8362, -47.8827) -> (88.8425, -47.8393) construction
  line L350 (88.8425, -47.8393) -> (88.8492, -47.7973) construction
  line L351 (88.8492, -47.7973) -> (88.8549, -47.7497) construction
  spline S76 degree 3 poles (88.8549, -47.7497) (89.0034, -46.5513) (89.4482, -47.5253) (89.5964, -48.1243) knots 0.482759 0.482759 0.482759 0.482759 0.5 0.5 0.5 0.5
  line L352 (88.8549, -47.7497) -> (89.0034, -46.5513) construction
  line L353 (89.0034, -46.5513) -> (89.4482, -47.5253) construction
  line L354 (89.4482, -47.5253) -> (89.5964, -48.1243) construction
  spline S77 degree 3 poles (89.5964, -48.1243) (89.6828, -48.4732) (89.794, -49.1756) (89.8719, -49.7034) knots 0.5 0.5 0.5 0.5 0.517241 0.517241 0.517241 0.517241
  line L355 (89.5964, -48.1243) -> (89.6828, -48.4732) construction
  line L356 (89.6828, -48.4732) -> (89.794, -49.1756) construction
  line L357 (89.794, -49.1756) -> (89.8719, -49.7034) construction
  spline S78 degree 3 poles (89.8719, -49.7034) (90.6371, -51.1649) (91.2855, -54.3291) (91.2862, -54.3322) knots 0.517241 0.517241 0.517241 0.517241 0.534483 0.534483 0.534483 0.534483
  line L358 (89.8719, -49.7034) -> (90.6371, -51.1649) construction
  line L359 (90.6371, -51.1649) -> (91.2862, -54.3322) construction
  line L360 (91.2862, -54.3322) -> (91.2862, -54.3322) construction
  spline S79 degree 3 poles (91.2862, -54.3322) (91.9417, -57.619) (91.0989, -57.4285) (90.3499, -59.8101) knots 0.534483 0.534483 0.534483 0.534483 0.551724 0.551724 0.551724 0.551724
  line L361 (91.2862, -54.3322) -> (91.9417, -57.619) construction
  line L362 (91.9417, -57.619) -> (91.0989, -57.4285) construction
  line L363 (91.0989, -57.4285) -> (90.3499, -59.8101) construction
  spline S80 degree 3 poles (90.3499, -59.8101) (89.6006, -62.1917) (90.2561, -63.8586) (91.2862, -66.9549) knots 0.551724 0.551724 0.551724 0.551724 0.568966 0.568966 0.568966 0.568966
  line L364 (90.3499, -59.8101) -> (89.6006, -62.1917) construction
  line L365 (89.6006, -62.1917) -> (90.2561, -63.8586) construction
  line L366 (90.2561, -63.8586) -> (91.2862, -66.9549) construction
  spline S81 degree 3 poles (91.2862, -66.9549) (92.316, -70.0505) (93.8595, -70.7646) (93.8611, -70.7653) knots 0.568966 0.568966 0.568966 0.568966 0.586207 0.586207 0.586207 0.586207
  line L367 (91.2862, -66.9549) -> (92.316, -70.0505) construction
  line L368 (92.316, -70.0505) -> (93.8611, -70.7653) construction
  line L369 (93.8611, -70.7653) -> (93.8611, -70.7653) construction
  spline S82 degree 3 poles (93.8611, -70.7653) (93.5803, -71.3844) (93.8608, -71.4796) (93.8611, -71.4796) knots 0.586207 0.586207 0.586207 0.586207 0.603448 0.603448 0.603448 0.603448
  line L370 (93.8611, -70.7653) -> (93.5803, -71.3844) construction
  line L371 (93.5803, -71.3844) -> (93.8611, -71.4796) construction
  line L372 (93.8611, -71.4796) -> (93.8611, -71.4796) construction
  line L373 (93.8611, -71.4796) -> (95.9679, -71.4796)
  spline S83 degree 3 poles (95.9679, -71.4796) (95.921, -70.67) (94.7985, -70.0512) (94.7974, -70.0505) knots 0.62069 0.62069 0.62069 0.62069 0.637931 0.637931 0.637931 0.637931
  line L374 (95.9679, -71.4796) -> (95.921, -70.67) construction
  line L375 (95.921, -70.67) -> (94.7974, -70.0505) construction
  line L376 (94.7974, -70.0505) -> (94.7974, -70.0505) construction
  spline S84 degree 3 poles (94.7974, -70.0505) (94.3762, -68.5265) (94.0952, -66.4804) (94.095, -66.4783) knots 0.637931 0.637931 0.637931 0.637931 0.655172 0.655172 0.655172 0.655172
  line L377 (94.7974, -70.0505) -> (94.3762, -68.5265) construction
  line L378 (94.3762, -68.5265) -> (94.095, -66.4783) construction
  line L379 (94.095, -66.4783) -> (94.095, -66.4783) construction
  spline S85 degree 3 poles (94.095, -66.4783) (93.0653, -62.3342) (94.562, -60.7642) (94.5635, -60.7626) knots 0.655172 0.655172 0.655172 0.655172 0.672414 0.672414 0.672414 0.672414
  line L380 (94.095, -66.4783) -> (93.0653, -62.3342) construction
  line L381 (93.0653, -62.3342) -> (94.5635, -60.7626) construction
  line L382 (94.5635, -60.7626) -> (94.5635, -60.7626) construction
  spline S86 degree 3 poles (94.5635, -60.7626) (96.8107, -58.9049) (97.4662, -57.238) (97.6066, -55.9994) (97.747, -54.7608) (98.3555, -54.6655) (99.011, -53.8559) knots 0.672414 0.672414 0.672414 0.672414 0.689655 0.689655 0.689655 0.706897 0.706897 0.706897 0.706897
  line L383 (94.5635, -60.7626) -> (96.8107, -58.9049) construction
  line L384 (96.8107, -58.9049) -> (97.4662, -57.238) construction
  line L385 (97.4662, -57.238) -> (97.6066, -55.9994) construction
  line L386 (97.6066, -55.9994) -> (97.747, -54.7608) construction
  line L387 (97.747, -54.7608) -> (98.3555, -54.6655) construction
  line L388 (98.3555, -54.6655) -> (99.011, -53.8559) construction
  spline S87 degree 3 poles (99.011, -53.8559) (99.6664, -53.0463) (100.1809, -51.2381) (100.1815, -51.2362) knots 0.706897 0.706897 0.706897 0.706897 0.724138 0.724138 0.724138 0.724138
  line L389 (99.011, -53.8559) -> (99.6664, -53.0463) construction
  line L390 (99.6664, -53.0463) -> (100.1815, -51.2362) construction
  line L391 (100.1815, -51.2362) -> (100.1815, -51.2362) construction
  spline S88 degree 3 poles (100.1815, -51.2362) (101.8671, -56.2375) (111.4082, -54.8099) (111.4178, -54.8084) knots 0.724138 0.724138 0.724138 0.724138 0.741379 0.741379 0.741379 0.741379
  line L392 (100.1815, -51.2362) -> (101.8671, -56.2375) construction
  line L393 (101.8671, -56.2375) -> (111.4178, -54.8084) construction
  line L394 (111.4178, -54.8084) -> (111.4178, -54.8084) construction
  spline S89 degree 3 poles (111.4178, -54.8084) (110.8717, -57.3488) (111.4178, -61.8738) (111.6521, -62.6676) knots 0.741379 0.741379 0.741379 0.741379 0.758621 0.758621 0.758621 0.758621
  line L395 (111.4178, -54.8084) -> (110.8717, -57.3488) construction
  line L396 (110.8717, -57.3488) -> (111.4178, -61.8738) construction
  line L397 (111.4178, -61.8738) -> (111.6521, -62.6676) construction
  spline S90 degree 3 poles (111.6521, -62.6676) (111.886, -63.4613) (112.5887, -65.0492) (112.8226, -67.193) knots 0.758621 0.758621 0.758621 0.758621 0.775862 0.775862 0.775862 0.775862
  line L398 (111.6521, -62.6676) -> (111.886, -63.4613) construction
  line L399 (111.886, -63.4613) -> (112.5887, -65.0492) construction
  line L400 (112.5887, -65.0492) -> (112.8226, -67.193) construction
  spline S91 degree 3 poles (112.8226, -67.193) (113.0568, -69.3365) (113.9921, -70.526) (113.9931, -70.5271) knots 0.775862 0.775862 0.775862 0.775862 0.793103 0.793103 0.793103 0.793103
  line L401 (112.8226, -67.193) -> (113.0568, -69.3365) construction
  line L402 (113.0568, -69.3365) -> (113.9931, -70.5271) construction
  line L403 (113.9931, -70.5271) -> (113.9931, -70.5271) construction
  spline S92 degree 3 poles (113.9931, -70.5271) (113.6029, -70.6859) (113.525, -71.7168) (113.525, -71.7178) knots 0.793103 0.793103 0.793103 0.793103 0.810345 0.810345 0.810345 0.810345
  line L404 (113.9931, -70.5271) -> (113.6029, -70.6859) construction
  line L405 (113.6029, -70.6859) -> (113.525, -71.7178) construction
  line L406 (113.525, -71.7178) -> (113.525, -71.7178) construction
  line L407 (113.525, -71.7178) -> (116.8023, -71.7178)
  line L408 (116.8023, -71.7178) -> (115.866, -70.289)
  spline S93 degree 3 poles (115.866, -70.289) (115.866, -70.2883) (115.9436, -69.5746) (115.3975, -66.7164) knots 0.844828 0.844828 0.844828 0.844828 0.862069 0.862069 0.862069 0.862069
  line L409 (115.866, -70.289) -> (115.866, -70.289) construction
  line L410 (115.866, -70.289) -> (115.9436, -69.5746) construction
  line L411 (115.9436, -69.5746) -> (115.3975, -66.7164) construction
  spline S94 degree 3 poles (115.3975, -66.7164) (114.8514, -63.8586) (115.7097, -63.0645) (116.3341, -60.5241) knots 0.862069 0.862069 0.862069 0.862069 0.87931 0.87931 0.87931 0.87931
  line L412 (115.3975, -66.7164) -> (114.8514, -63.8586) construction
  line L413 (114.8514, -63.8586) -> (115.7097, -63.0645) construction
  line L414 (115.7097, -63.0645) -> (116.3341, -60.5241) construction
  spline S95 degree 3 poles (116.3341, -60.5241) (116.9582, -57.9841) (116.9582, -55.285) (117.5043, -55.0465) knots 0.87931 0.87931 0.87931 0.87931 0.896552 0.896552 0.896552 0.896552
  line L415 (116.3341, -60.5241) -> (116.9582, -57.9841) construction
  line L416 (116.9582, -57.9841) -> (116.9582, -55.285) construction
  line L417 (116.9582, -55.285) -> (117.5043, -55.0465) construction
  spline S96 degree 3 poles (117.5043, -55.0465) (118.0507, -54.8084) (118.9091, -53.9353) (119.1433, -53.3797) knots 0.896552 0.896552 0.896552 0.896552 0.913793 0.913793 0.913793 0.913793
  line L418 (117.5043, -55.0465) -> (118.0507, -54.8084) construction
  line L419 (118.0507, -54.8084) -> (118.9091, -53.9353) construction
  line L420 (118.9091, -53.9353) -> (119.1433, -53.3797) construction
  spline S97 degree 3 poles (119.1433, -53.3797) (119.3772, -52.824) (120.0796, -50.6806) (122.6545, -48.1402) knots 0.913793 0.913793 0.913793 0.913793 0.931034 0.931034 0.931034 0.931034
  line L421 (119.1433, -53.3797) -> (119.3772, -52.824) construction